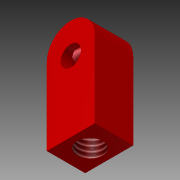
# Autodesk Inventor part: HoseBarbAddOn
Saved by Autodesk Inventor 2012 SP1 (Build 160190100, 190)
## iProperties
Created: 2010-03-29
Part Number: HoseBarbAddOn
Document SubType Name: Modeling
Designer: rconnaug
Density: 2.71 g/cm^3
Material: Aluminum-6061
Mass: 1.36249 g
Surface Area: 6.42833 cm^2
Volume: 0.502763 cm^3
Author: rconnaug
Autodesk Inventor part; units mm, degrees
ref_plane "YZ Plane" through (0, 0, 0) normal (1, 0, 0) x (0, 1, 0)
ref_plane "XZ Plane" through (0, 0, 0) normal (0, 1, 0) x (-1, 0, 0)
ref_plane "XY Plane" through (0, 0, 0) normal (0, 0, 1) x (1, 0, 0)
sketch "Sketch1" plane through (0, 0, 0) normal (0, 0, 1) x (1, 0, 0)
  line L0 (-5.25, 0) -> (5.25, 0) projected
  line L1 (0, -3.15) -> (0, 18.9) projected
  line L2 (3.75, 12) -> (3.75, 0)
  line L3 (3.75, 0) -> (-3.75, 0)
  line L4 (-3.75, 0) -> (-3.75, 12)
  arc A0 (3.75, 12) -> (-3.75, 12) centre (0, 12) ccw
  point P0 (0, 0)
  dimension "d0" = 7.5
  dimension "d1" = 12
  constraints: 6 end point, 2 point on circle, 2 tangent, 2 vertical, 1 centre point, 1 collinear, 1 parallel, 1 point on line
  measures "d0" distance between parallel lines of L2 L4
  measures "d1" distance from line of L3 A0.centre
extrude "Extrusion1" add sketch "Sketch1" along normal blind 6
sketch "Sketch2" plane through (-3.75, 0, 0) normal (0, -1, 0) x (1, 0, 0)
  line L0 (0, 0) -> (7.5, 0) projected
  line L1 (7.5, 0) -> (7.5, 6) projected
  point P0 (0, 6)
  point P1 (3.75, 0)
  point P2 (3.75, 3)
  dimension "d4" = 7.5
  dimension "d5" = 6
  dimension "d6" = 3.75
  dimension "d7" = 3
  measures "d4" distance of L1.end point (0, 6)
  measures "d5" distance of L0.end L1.end
  measures "d6" distance from line of L1 point (3.75, 3)
  measures "d7" distance from line of L0 point (3.75, 3)
hole "Hole1" at (0, 0, 3) direction (0, 1, 0) diameter 3.962 depth 12.5 tip angle 118 thread size "10-32 UNF" class "2B" standard "ANSI Unified Screw Threads"
sketch "Sketch3" plane through (0, 0, 0) normal (0, 0, -1) x (-1, 0, 0)
  arc A0 (3.75, 12) -> (-3.75, 12) centre (0, 12) ccw projected
  circle A1 centre (0, 11) radius 1.5875
  line L0 (0, -3.15) -> (0, 18.9) projected
  point P0 (0, 0)
  dimension "d15" = 3.175
  dimension "d16" = 1
  constraints: 1 centre point, 1 point on line
  measures "d15" diameter of A1
  measures "d16" distance of A0.centre A1.centre
extrude "Extrusion2" cut sketch "Sketch3" against normal blind 2
equation "\"d6\" = 0.5 * d4"
equation "\"d7\" = 0.5 * d5"
body "Solid1"
